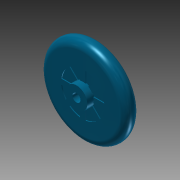
# Autodesk Inventor part: 13-0003
Saved by Autodesk Inventor 2015 SP1 (Build 190203100, 203)
## iProperties
Category: Caster Wheel Kit
Company: Autodesk Inc.
Created: 2014-11-30
Part Number: 13-0003
Material: Polystyrene, High Impact
Document SubType Name: Modeling
Designer: Matrix
Density: 1.022 g/cm^3
Appearance: Sky Blue Dark
Catalog Web Link: http://matrixrobotics.com/
Vendor: Matrix
Author: Autodesk Inc.
Autodesk Inventor part; units mm, degrees
ref_plane "YZ Plane" through (0, 0, 0) normal (1, 0, 0) x (0, 1, 0)
ref_plane "XZ Plane" through (0, 0, 0) normal (0, 1, 0) x (-1, 0, 0)
sketch "Sketch1" plane through (0, 0, 0) normal (0, 1, 0) x (-1, 0, 0)
  circle A0 centre (0, 0) radius 24
  dimension "d0" = 48
  constraints: 1 centre point, 1 coincident
  measures "d0" diameter of A0
extrude "Extrusion1" add sketch "Sketch1" against normal blind 8
fillet "Fillet1" radius 4 2 edges at (24, 0, 0) (24, -8, 0)
sketch "Sketch2" plane through (0, -8, 0) normal (0, -1, 0) x (1, 0, 0)
  circle A0 centre (0, 0) radius 12
  line L0 (-7.3581, 9.4794) -> (-3.0473, 5.1686)
  arc A1 (-1.5, 5.8095) -> (-3.0473, 5.1686) centre (0, 0) ccw
  line L1 (-1.5, 5.8095) -> (-1.5, 11.9059)
  arc A2 (-1.5, 11.9059) -> (-7.3581, 9.4794) centre (0, 0) ccw
  line L2 (3.0473, 5.1686) -> (7.3581, 9.4794)
  arc A3 (7.3581, 9.4794) -> (1.5, 11.9059) centre (0, 0) ccw
  line L3 (1.5, 11.9059) -> (1.5, 5.8095)
  arc A4 (3.0473, 5.1686) -> (1.5, 5.8095) centre (0, 0) ccw
  line L4 (9.4794, 7.3581) -> (5.1686, 3.0473)
  arc A5 (5.8095, 1.5) -> (5.1686, 3.0473) centre (0, 0) ccw
  line L5 (5.8095, 1.5) -> (11.9059, 1.5)
  arc A6 (11.9059, 1.5) -> (9.4794, 7.3581) centre (0, 0) ccw
  line L6 (11.9059, -1.5) -> (5.8095, -1.5)
  arc A7 (5.1686, -3.0473) -> (5.8095, -1.5) centre (0, 0) ccw
  line L7 (5.1686, -3.0473) -> (9.4794, -7.3581)
  arc A8 (9.4794, -7.3581) -> (11.9059, -1.5) centre (0, 0) ccw
  line L8 (7.3581, -9.4794) -> (3.0473, -5.1686)
  arc A9 (1.5, -5.8095) -> (3.0473, -5.1686) centre (0, 0) ccw
  line L9 (1.5, -5.8095) -> (1.5, -11.9059)
  arc A10 (1.5, -11.9059) -> (7.3581, -9.4794) centre (0, 0) ccw
  line L10 (-3.0473, -5.1686) -> (-7.3581, -9.4794)
  arc A11 (-7.3581, -9.4794) -> (-1.5, -11.9059) centre (0, 0) ccw
  line L11 (-1.5, -11.9059) -> (-1.5, -5.8095)
  arc A12 (-3.0473, -5.1686) -> (-1.5, -5.8095) centre (0, 0) ccw
  line L12 (-9.4794, -7.3581) -> (-5.1686, -3.0473)
  arc A13 (-5.8095, -1.5) -> (-5.1686, -3.0473) centre (0, 0) ccw
  line L13 (-5.8095, -1.5) -> (-11.9059, -1.5)
  arc A14 (-11.9059, -1.5) -> (-9.4794, -7.3581) centre (0, 0) ccw
  line L14 (-5.1686, 3.0473) -> (-9.4794, 7.3581)
  arc A15 (-9.4794, 7.3581) -> (-11.9059, 1.5) centre (0, 0) ccw
  line L15 (-11.9059, 1.5) -> (-5.8095, 1.5)
  arc A16 (-5.1686, 3.0473) -> (-5.8095, 1.5) centre (0, 0) ccw
  circle A17 centre (0, 0) radius 6
  circle A18 centre (0, 0) radius 2.1
  point P0 (-6, 0)
  constraints: 32 end point, 32 point on circle, 19 centre point
extrude "Extrusion2" cut sketch "Sketch2" against normal blind 0.5 contours L5 A5 L4 A0 | A0 L7 A7 L6 | L2 A4 L3 A0 | A0 L9 A9 L8 | L1 A1 L0 A0 | A0 L10 A12 L11 | L14 A16 L15 A0 | A0 L13 A13 L12
sketch "Sketch3" plane through (0, -8, 0) normal (0, -1, 0) x (1, 0, 0)
  arc A0 (3.0473, 5.1686) -> (1.5, 5.8095) centre (0, 0) ccw projected
  circle A1 centre (0, 0) radius 6
  constraints: 1 centre point, 1 coincident
extrude "Extrusion3" add sketch "Sketch3" along normal blind 3.5
ref_plane "Work Plane1" through (0, -4, 0) normal (0, -1, 0) x (1, 0, 0)
mirror "Mirror1" about plane through (0, -4, 0) normal (0, -1, 0) of "Extrusion2", "Extrusion3"
sketch "Sketch4" plane through (0, -11.5, 0) normal (0, -1, 0) x (1, 0, 0)
  point P0 (0, 0)
hole "Hole1" at (0, -11.5, 0) direction (0, 1, 0) diameter 4.5 end through all
body "Solid1"
